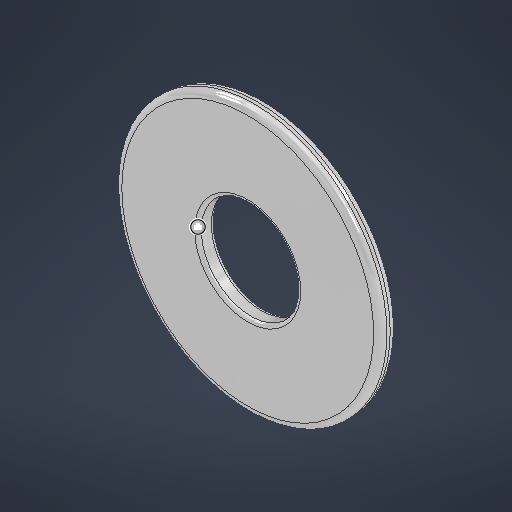
# Autodesk Inventor part: Anilha_M3
Saved by Autodesk Inventor 2025.2 (Build 292293000, 293)
## iProperties
Created: 2025-05-28
Part Number: Anilha_M3
Material: Generic
Document SubType Name: Modeling
Designer: Tiago
Density: 1 g/cm^3
Appearance: Aluminum - Dark
Author: Tiago
Autodesk Inventor part; units mm, degrees
ref_plane "YZ Plane" through (0, 0, 0) normal (1, 0, 0) x (0, 1, 0)
ref_plane "XZ Plane" through (0, 0, 0) normal (0, 1, 0) x (-1, 0, 0)
ref_plane "XY Plane" through (0, 0, 0) normal (0, 0, 1) x (1, 0, 0)
sketch "Sketch1" plane through (0, 0, 0) normal (0, 0, 1) x (1, 0, 0)
  circle A0 centre (0, 0) radius 1.5
  circle A1 centre (0, 0) radius 4
  dimension "Di" = 3
  dimension "D" = 8
  constraints: 2 centre point, 2 coincident
  measures "Di" diameter of A0
  measures "D" diameter of A1
extrude "Extrusion1" add sketch "Sketch1" along normal mid plane 0.5
fillet "Fillet1" radius 0.2 2 edges at (-4, 0, 0.25) (-4, 0, -0.25)
fillet "Fillet2" radius 0.1 2 edges at (-1.5, 0, 0.25) (-1.5, 0, -0.25)
body "Solid1"
